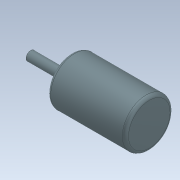
# Autodesk Inventor part: Motor
Saved by Autodesk Inventor 2021 (Build 250183000, 183)
## iProperties
Created: 2021-08-29
Part Number: Motor
Material: Iron, Cast
Document SubType Name: Modeling
Designer: digge
Density: 7.15 g/cm^3
Appearance: Lead
Author: digge
Autodesk Inventor part; units mm, degrees
ref_plane "YZ Plane" through (0, 0, 0) normal (1, 0, 0) x (0, 1, 0)
ref_plane "XZ Plane" through (0, 0, 0) normal (0, 1, 0) x (-1, 0, 0)
ref_plane "XY Plane" through (0, 0, 0) normal (0, 0, 1) x (1, 0, 0)
sketch "Sketch1" plane through (0, 0, 0) normal (0, 0, 1) x (1, 0, 0)
  line L0 (-41.8167, 33.637) -> (-16.7167, 33.637)
  line L1 (-16.7167, 33.637) -> (-16.7167, 25.937)
  line L2 (-16.7167, 25.937) -> (-39.8, 25.937)
  line L3 (-39.8, 25.937) -> (-42.3, 25.937)
  line L4 (-42.3, 25.937) -> (-54.9667, 25.937)
  line L5 (-54.9667, 25.937) -> (-54.9667, 27.437)
  line L6 (-54.9667, 27.437) -> (-43.4167, 27.437)
  line L7 (-43.4167, 27.437) -> (-43.4167, 29.012)
  line L8 (-43.4167, 29.012) -> (-41.8167, 29.012)
  line L9 (-41.8167, 29.012) -> (-41.8167, 33.637)
  point P0 (0, 0)
  dimension "d0" = 1.5
  dimension "d1" = 7.7
  dimension "d2" = 1.6
  dimension "d3" = 25.1
  dimension "d4" = 11.55
  dimension "d5" = 3.075
  constraints: 20 end point, 6 perpendicular, 2 point on line, 1 horizontal, 1 parallel
  measures "d0" distance of L4.end L5.end
  measures "d1" distance between parallel lines of L2 L0
  measures "d2" distance of L7.end L8.end
  measures "d3" distance of L0.start L0.end
  measures "d4" distance of L5.end L6.end
  measures "d5" distance from line of L3.end L8
revolve "Revolution1" add sketch "Sketch1" angle 360 about axis through (-16.7167, 25.937, 0) along (-1, 0, 0)
fillet "Fillet1" radius 1 2 edges at (-41.8167, 18.237, 0) (-43.4167, 22.862, 0)
fillet "Fillet2" radius 1 1 edges at (-16.7167, 18.237, 0)
body "Solid1"
